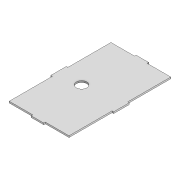
# Autodesk Inventor part: 본체 뚜껑 레이저 수정
Saved by Autodesk Inventor 2020 (Build 240168000, 168)
## iProperties
Created: 2022-08-25
Part Number: 본체 뚜껑 레이저 수정
Material: 일반
Document SubType Name: Modeling
Designer: 박연호
Density: 1 g/cm^3
Appearance: 기본값
Author: 박연호
Autodesk Inventor part; units mm, degrees
ref_plane "YZ Plane" through (0, 0, 0) normal (1, 0, 0) x (0, 1, 0)
ref_plane "XZ Plane" through (0, 0, 0) normal (0, 1, 0) x (-1, 0, 0)
ref_plane "XY Plane" through (0, 0, 0) normal (0, 0, 1) x (1, 0, 0)
sketch "스케치1" plane through (0, 0, 0) normal (0, 1, 0) x (-1, 0, 0)
  line L0 (-60, 100) -> (60, 100)
  line L1 (60, 100) -> (60, -100)
  line L2 (60, -100) -> (-60, -100)
  line L3 (-60, -100) -> (-60, 100)
  line L4 (-60, 100) -> (60, -100) construction
  line L5 (60, 100) -> (-60, -100) construction
  point P0 (0, 0)
  dimension "d0" = 200
  dimension "d1" = 120
  constraints: 12 end point, 2 midpoint, 2 parallel, 1 horizontal, 1 perpendicular
  measures "d0" distance of L0.end L1.end
  measures "d1" distance of L1.end L2.end
extrude "돌출1" add sketch "스케치1" along normal blind 3
sketch "스케치2" plane through (0, 3, 0) normal (0, 1, 0) x (1, 0, 0)
  circle A0 centre (-15, -1) radius 10
  line L0 (-60, 100) -> (-60, -100) projected
  line L1 (60, 100) -> (-60, 100) projected
  point P0 (0, 0)
  dimension "d4" = 20
  dimension "d5" = 45
  dimension "d6" = 101
  constraints: 1 centre point
  measures "d4" diameter of A0
  measures "d5" distance from line of A0.centre L0
  measures "d6" distance from line of A0.centre L1
extrude "돌출2" cut sketch "스케치2" against normal through all
sketch "스케치3" plane through (0, 3, 0) normal (0, 1, 0) x (1, 0, 0)
  line L0 (-60, 15) -> (-57, 15)
  line L1 (-57, 15) -> (-57, 100)
  line L2 (-57, 100) -> (-60, 100)
  line L3 (-60, 100) -> (-60, 15)
  line L4 (-60, 100) -> (-60, -100) projected
  line L5 (60, 100) -> (-60, 100) projected
  line L6 (-60, 100) -> (-60, -100) projected
  line L7 (-60, 0) -> (60, 0)
  line L8 (60, -100) -> (60, 100) projected
  line L9 (60, 100) -> (-60, 100) projected
  line L10 (0, 100) -> (0, -100)
  line L11 (-60, -100) -> (60, -100) projected
  line L12 (-60, -15) -> (-57, -15)
  line L13 (-57, -15) -> (-57, -100)
  line L14 (-57, -100) -> (-60, -100)
  line L15 (-60, -100) -> (-60, -15)
  line L16 (60, 15) -> (57, 15)
  line L17 (57, 15) -> (57, 100)
  line L18 (57, 100) -> (60, 100)
  line L19 (60, 100) -> (60, 15)
  line L20 (60, 100) -> (60, -100)
  line L21 (60, 100) -> (60, -100)
  line L22 (60, -15) -> (57, -15)
  line L23 (57, -15) -> (57, -100)
  line L24 (57, -100) -> (60, -100)
  line L25 (60, -100) -> (60, -15)
  point P0 (0, 0)
  point P1 (-60, -100)
  point P2 (60, -100)
  dimension "d9" = 85
  dimension "d10" = 3
  constraints: 40 end point, 16 symmetric about line, 4 midpoint, 2 collinear, 2 parallel, 1 horizontal, 1 perpendicular
  measures "d9" distance between parallel lines of L2 L0
  measures "d10" distance between parallel lines of L1 L3
extrude "돌출3" cut sketch "스케치3" against normal through all contours L3 L2 L1 L0 | L12 L13 L11 L4 | L5 L8 L16 L17 | L8 L11 L23 L22
sketch "스케치4" plane through (0, 3, 0) normal (0, 1, 0) x (1, 0, 0)
  line L0 (-57, -100) -> (57, -100) projected
  line L1 (57, -100) -> (12, -100)
  line L2 (12, -100) -> (12, -97)
  line L3 (12, -97) -> (57, -97)
  line L4 (57, -97) -> (57, -100)
  line L5 (0, -100) -> (0, 100)
  line L6 (57, 100) -> (-57, 100) projected
  line L7 (-59.774, 0) -> (60, 0)
  line L8 (60, -15) -> (60, 15) projected
  line L9 (57, 100) -> (12, 100)
  line L10 (12, 100) -> (12, 97)
  line L11 (12, 97) -> (57, 97)
  line L12 (57, 97) -> (57, 100)
  line L13 (-57, -100) -> (-12, -100)
  line L14 (-12, -100) -> (-12, -97)
  line L15 (-12, -97) -> (-57, -97)
  line L16 (-57, -97) -> (-57, -100)
  line L17 (-57, 100) -> (-12, 100)
  line L18 (-12, 100) -> (-12, 97)
  line L19 (-12, 97) -> (-57, 97)
  line L20 (-57, 97) -> (-57, 100)
  point P0 (0, 0)
  point P1 (-12, 100)
  point P2 (12, 100)
  dimension "d13" = 3
  dimension "d14" = 45
  constraints: 36 end point, 9 symmetric about line, 3 midpoint, 2 parallel, 1 horizontal, 1 perpendicular
  measures "d13" distance of L3.end L0.end
  measures "d14" distance of L2.end L3.end
extrude "돌출4" cut sketch "스케치4" against normal through all
